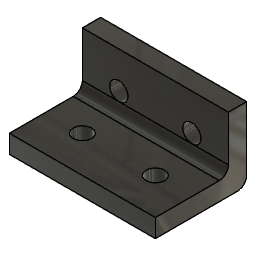
ClamporMount Bracket (Autodesk Fusion 360 design; units mm, degrees)
Autodesk Fusion 360 part; units mm, degrees
sketch "Sketch1" plane through (0, 0, 0) normal (0, 1, 0) x (1, 0, 0)
  line L0 (50.8, 25.4) -> (-50.8, 25.4)
  line L1 (-50.8, 25.4) -> (-50.8, -25.4)
  line L2 (-50.8, -25.4) -> (50.8, -25.4)
  line L3 (50.8, -25.4) -> (50.8, 25.4)
  line L4 (0, 0) -> (25.4, 0) construction
  line L5 (0, 0) -> (-25.4, 0) construction
  circle A0 centre (-25.4, 0) radius 6.35
  circle A1 centre (25.4, 0) radius 6.35
  dimension "d3" = 101.6
  dimension "d4" = 50.8
  dimension "d5" = 25.4
  dimension "d7" = 12.7
  dimension "d8" = 12.7
  constraint horizontal L0
  constraint perpendicular L0 L1
  constraint parallel L0 L2
  constraint parallel L1 L3
  constraint coincident L4.start L5.start
  constraint horizontal L4
  constraint parallel L4 L5
  constraint coincident L5.end A0.centre
  constraint coincident L4.end A1.centre
  measures "d3" distance of L1.end L2.end
  measures "d4" distance of L0.end L1.end
  measures "d5" distance of L4.start L4.end
  measures "d7" diameter of A0
  measures "d8" diameter of A1
extrude "Extrude1" add sketch "Sketch1" along normal blind 12.7 makes body 1
sketch "Sketch2" plane through (0, 0, 0) normal (0, -1, 0) x (1, 0, 0)
  circle A0 centre (-25.4, 0) radius 6.35
  circle A1 centre (25.4, 0) radius 6.35
  line L0 (50.8, -25.4) -> (50.8, 25.4)
  line L1 (50.8, 25.4) -> (-50.8, 25.4)
  line L2 (-50.8, 25.4) -> (-50.8, -25.4)
  line L3 (-50.8, -25.4) -> (50.8, -25.4)
  line L4 (-50.8, -25.4) -> (50.8, -25.4)
  line L5 (50.8, -25.4) -> (50.8, -12.7)
  line L6 (50.8, -12.7) -> (-50.8, -12.7)
  line L7 (-50.8, -12.7) -> (-50.8, -25.4)
  dimension "d11" = 101.6
  dimension "d12" = 12.7
  constraint horizontal L4
  constraint vertical L5
  constraint horizontal L6
  constraint vertical L7
  constraint coincident L2.end L3.start
  measures "d11" distance of L2.end L0.start
  measures "d12" distance of L0.start L5.end
extrude "Extrude2" add sketch "Sketch2" along normal blind 50.8 contours L0 L2 L3 L4 L5 L6 L7 bodies 1
sketch "Sketch3" plane through (0, 0, -12.7) normal (0, 0, 1) x (-1, 0, 0)
  line L0 (-50.8, 0) -> (50.8, 0)
  line L1 (50.8, 0) -> (50.8, 50.8)
  line L2 (50.8, 50.8) -> (-50.8, 50.8)
  line L3 (-50.8, 50.8) -> (-50.8, 0)
  line L4 (0, 0) -> (0, 50.8) construction
  line L5 (0, 25.4) -> (-25.4, 25.4) construction
  line L6 (0, 25.4) -> (25.4, 25.4) construction
  circle A0 centre (25.4, 25.4) radius 6.35
  circle A1 centre (-25.4, 25.4) radius 6.35
  dimension "d15" = 25.4
  dimension "d16" = 25.4
  dimension "d17" = 12.7
  dimension "d18" = 12.7
  constraint coincident L4.start origin
  constraint midpoint L2 L4.end
  constraint midpoint L4 L5.start
  constraint perpendicular L4 L5
  constraint perpendicular L4 L6
  constraint coincident L6.end A0.centre
  constraint coincident L5.end A1.centre
  measures "d15" distance of L5.start L5.end
  measures "d16" distance of L5.start L6.end
  measures "d17" diameter of A0
  measures "d18" diameter of A1
extrude "Extrude3" cut sketch "Sketch3" against normal blind 43.18 contours A0 | A1 bodies 1
fillet "Fillet1" radius 6.35 2 edges at (0, 0, -12.7) (0, 12.7, -25.4) on bodies 1
copy_body "Body->Comp1" bodies 1 removing the originals makes body 2 in component "Clamp/Mount Bracket"
component "Clamp/Mount Bracket" placed x (1, 0, 0) y (0, 1, 0) z (0, 0, 1) at (0, 0, 0)
equation "d7 = ( 1 / 2 ) * 1 in"
equation "d8 = ( 1 / 2 ) * 1 in"
equation "d9 = ( 1 / 2 ) * 1 in"
equation "d17 = ( 1 / 2 ) * 1 in"
equation "d18 = ( 1 / 2 ) * 1 in"
equation "d22 = ( 1 / 4 ) * 1 in"
